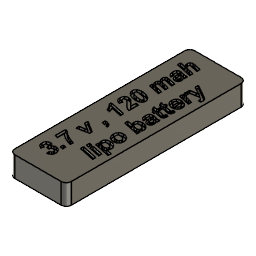
Battery (Autodesk Fusion 360 design; units mm, degrees)
part number: 2026-07-18-00-20-30-894
Autodesk Fusion 360 part; units mm, degrees
sketch "Sketch1" plane through (0, 0, 0) normal (0, 0, 1) x (1, 0, 0)
  line L0 (-49, 45) -> (-40, 45)
  line L1 (-39, 44) -> (-39, 11)
  line L2 (-40, 10) -> (-49, 10)
  line L3 (-50, 11) -> (-50, 44)
  arc A0 (-49, 45) -> (-50, 44) centre (-49, 44) ccw
  arc A1 (-39, 44) -> (-40, 45) centre (-40, 44) ccw
  arc A2 (-40, 10) -> (-39, 11) centre (-40, 11) ccw
  arc A3 (-50, 11) -> (-49, 10) centre (-49, 11) ccw
  point P0 (-50, 45)
  point P1 (-39, 45)
  point P2 (-50, 10)
  dimension "d3" = 11
  dimension "d4" = 35
  dimension "d5" = 1
  constraint perpendicular L0 L1
  constraint parallel L0 L2
  constraint parallel L1 L3
  constraint horizontal L0
  constraint coincident P0 L0
  constraint coincident P0 L3
  constraint tangent L0 A0
  constraint tangent L3 A0
  constraint coincident P1 L0
  constraint coincident P1 L1
  constraint tangent L0 A1
  constraint tangent L1 A1
  constraint equal A0 A1
  constraint tangent L1 A2
  constraint tangent L2 A2
  constraint equal A0 A2
  constraint coincident P2 L2
  constraint coincident P2 L3
  constraint tangent L2 A3
  constraint tangent L3 A3
  constraint equal A0 A3
  measures "d3" distance of P0 P1
  measures "d4" distance of P0 P2
  measures "d5" radius of A0
extrude "Extrude1" add sketch "Sketch1" along normal blind 4
sketch "Sketch2" plane through (0, 0, 4) normal (0, 0, 1) x (-1, 0, 0)
  arc A0 (49, -45) -> (50, -44) centre (49, -44) ccw
  line L0 (50, -44) -> (50, -11)
  arc A1 (50, -11) -> (49, -10) centre (49, -11) ccw
  line L1 (49, -10) -> (40, -10)
  arc A2 (40, -10) -> (39, -11) centre (40, -11) ccw
  line L2 (39, -11) -> (39, -44)
  arc A3 (39, -44) -> (40, -45) centre (40, -44) ccw
  line L3 (40, -45) -> (49, -45)
  line L4 (46.1248, -13.354) -> (46.1924, -13.9168)
  spline S0 degree 2 poles (46.1924, -13.9168) (45.9529, -13.9516) (45.8608, -14.0426) knots 0 0 0 1 1 1
  spline S1 degree 2 poles (45.8608, -14.0426) (45.7688, -14.1337) (45.7688, -14.2851) knots 0 0 0 1 1 1
  spline S2 degree 2 poles (45.7688, -14.2851) (45.7688, -14.4857) (45.9038, -14.6177) knots 0 0 0 1 1 1
  spline S3 degree 2 poles (45.9038, -14.6177) (46.0389, -14.7497) (46.2497, -14.7497) knots 0 0 0 1 1 1
  spline S4 degree 2 poles (46.2497, -14.7497) (46.4338, -14.7497) (46.5413, -14.6432) knots 0 0 0 1 1 1
  spline S5 degree 2 poles (46.5413, -14.6432) (46.6487, -14.5368) (46.6487, -14.3568) knots 0 0 0 1 1 1
  spline S6 degree 2 poles (46.6487, -14.3568) (46.6487, -14.3117) (46.6405, -14.2626) knots 0 0 0 1 1 1
  line L5 (46.6405, -14.2626) -> (47.1296, -14.3649)
  spline S7 degree 2 poles (47.1296, -14.3649) (47.1255, -14.3956) (47.1255, -14.4243) knots 0 0 0 1 1 1
  spline S8 degree 2 poles (47.1255, -14.4243) (47.1255, -14.6596) (47.2452, -14.7824) knots 0 0 0 1 1 1
  spline S9 degree 2 poles (47.2452, -14.7824) (47.3649, -14.9052) (47.5696, -14.9052) knots 0 0 0 1 1 1
  spline S10 degree 2 poles (47.5696, -14.9052) (47.7149, -14.9052) (47.7988, -14.8223) knots 0 0 0 1 1 1
  spline S11 degree 2 poles (47.7988, -14.8223) (47.8827, -14.7394) (47.8827, -14.6044) knots 0 0 0 1 1 1
  spline S12 degree 2 poles (47.8827, -14.6044) (47.8827, -14.4775) (47.7896, -14.3772) knots 0 0 0 1 1 1
  spline S13 degree 2 poles (47.7896, -14.3772) (47.6965, -14.2769) (47.4714, -14.2176) knots 0 0 0 1 1 1
  line L6 (47.4714, -14.2176) -> (47.5778, -13.6814)
  spline S14 degree 2 poles (47.5778, -13.6814) (47.9093, -13.7838) (48.0873, -13.9659) knots 0 0 0 1 1 1
  spline S15 degree 2 poles (48.0873, -13.9659) (48.3533, -14.2422) (48.3533, -14.6453) knots 0 0 0 1 1 1
  spline S16 degree 2 poles (48.3533, -14.6453) (48.3533, -15.0587) (48.1231, -15.2735) knots 0 0 0 1 1 1
  spline S17 degree 2 poles (48.1231, -15.2735) (47.8929, -15.4884) (47.5716, -15.4884) knots 0 0 0 1 1 1
  spline S18 degree 2 poles (47.5716, -15.4884) (47.3383, -15.4884) (47.1501, -15.3513) knots 0 0 0 1 1 1
  spline S19 degree 2 poles (47.1501, -15.3513) (46.9618, -15.2142) (46.8738, -14.9748) knots 0 0 0 1 1 1
  spline S20 degree 2 poles (46.8738, -14.9748) (46.7735, -15.1651) (46.6139, -15.2551) knots 0 0 0 1 1 1
  spline S21 degree 2 poles (46.6139, -15.2551) (46.4543, -15.3452) (46.2804, -15.3452) knots 0 0 0 1 1 1
  spline S22 degree 2 poles (46.2804, -15.3452) (45.9488, -15.3452) (45.6705, -15.1098) knots 0 0 0 1 1 1
  spline S23 degree 2 poles (45.6705, -15.1098) (45.2899, -14.7885) (45.2899, -14.281) knots 0 0 0 1 1 1
  spline S24 degree 2 poles (45.2899, -14.281) (45.2899, -13.9004) (45.5078, -13.6538) knots 0 0 0 1 1 1
  spline S25 degree 2 poles (45.5078, -13.6538) (45.7258, -13.4072) (46.1248, -13.354) knots 0 0 0 1 1 1
  line L7 (45.9079, -15.7749) -> (45.9079, -16.3561)
  line L8 (45.9079, -16.3561) -> (45.3411, -16.2374)
  line L9 (45.3411, -16.2374) -> (45.3411, -15.6562)
  line L10 (45.3411, -15.6562) -> (45.9079, -15.7749)
  line L11 (47.7578, -17.0703) -> (48.3001, -17.1828)
  line L12 (48.3001, -17.1828) -> (48.3001, -19.1617)
  line L13 (48.3001, -19.1617) -> (47.8827, -19.0737)
  spline S26 degree 2 poles (47.8827, -19.0737) (47.7312, -18.8854) (47.4274, -18.6583) knots 0 0 0 1 1 1
  spline S27 degree 2 poles (47.4274, -18.6583) (47.1235, -18.4311) (46.748, -18.2377) knots 0 0 0 1 1 1
  spline S28 degree 2 poles (46.748, -18.2377) (46.3724, -18.0443) (46.0348, -17.9216) knots 0 0 0 1 1 1
  spline S29 degree 2 poles (46.0348, -17.9216) (45.5682, -17.7517) (45.3411, -17.7108) knots 0 0 0 1 1 1
  line L14 (45.3411, -17.7108) -> (45.3411, -17.1521)
  spline S30 degree 2 poles (45.3411, -17.1521) (45.5662, -17.189) (45.9591, -17.3261) knots 0 0 0 1 1 1
  spline S31 degree 2 poles (45.9591, -17.3261) (46.442, -17.4939) (46.8922, -17.7456) knots 0 0 0 1 1 1
  spline S32 degree 2 poles (46.8922, -17.7456) (47.3424, -17.9973) (47.7578, -18.3533) knots 0 0 0 1 1 1
  line L15 (47.7578, -18.3533) -> (47.7578, -17.0703)
  line L16 (45.3411, -21.3861) -> (45.3411, -20.8806)
  line L17 (45.3411, -20.8806) -> (47.5143, -20.4447)
  line L18 (47.5143, -20.4447) -> (47.5143, -21.0218)
  line L19 (47.5143, -21.0218) -> (46.5668, -21.1753)
  spline S33 degree 2 poles (46.5668, -21.1753) (46.1821, -21.2387) (46.0553, -21.251) knots 0 0 0 1 1 1
  spline S34 degree 2 poles (46.0553, -21.251) (46.09, -21.2674) (46.3203, -21.3932) knots 0 0 0 1 1 1
  spline S35 degree 2 poles (46.3203, -21.3932) (46.5505, -21.5191) (46.5975, -21.5478) knots 0 0 0 1 1 1
  line L20 (46.5975, -21.5478) -> (47.5143, -22.088)
  line L21 (47.5143, -22.088) -> (47.5143, -22.7224)
  line L22 (47.5143, -22.7224) -> (45.3411, -21.3861)
  line L23 (45.9079, -23.9256) -> (45.9079, -24.5171)
  line L24 (45.9079, -24.5171) -> (45.4393, -24.4188)
  spline S36 degree 2 poles (45.4393, -24.4188) (45.0341, -24.3349) (44.8653, -24.1497) knots 0 0 0 1 1 1
  spline S37 degree 2 poles (44.8653, -24.1497) (44.6965, -23.9645) (44.6903, -23.6699) knots 0 0 0 1 1 1
  line L25 (44.6903, -23.6699) -> (44.9625, -23.7271)
  spline S38 degree 2 poles (44.9625, -23.7271) (44.9952, -23.8745) (45.0802, -23.9553) knots 0 0 0 1 1 1
  spline S39 degree 2 poles (45.0802, -23.9553) (45.1651, -24.0362) (45.3411, -24.075) knots 0 0 0 1 1 1
  line L26 (45.3411, -24.075) -> (45.3411, -23.8049)
  line L27 (45.3411, -23.8049) -> (45.9079, -23.9256)
  line L28 (47.0641, -26.4529) -> (47.588, -26.5634)
  spline S40 degree 2 poles (47.588, -26.5634) (47.9195, -27.3226) (48.3595, -27.7381) knots 0 0 0 1 1 1
  line L29 (48.3595, -27.7381) -> (48.3595, -28.0962)
  line L30 (48.3595, -28.0962) -> (45.3411, -27.4638)
  line L31 (45.3411, -27.4638) -> (45.3411, -26.8724)
  line L32 (45.3411, -26.8724) -> (47.4202, -27.3083)
  spline S41 degree 2 poles (47.4202, -27.3083) (47.3015, -27.1241) (47.2033, -26.8837) knots 0 0 0 1 1 1
  spline S42 degree 2 poles (47.2033, -26.8837) (47.105, -26.6432) (47.0641, -26.4529) knots 0 0 0 1 1 1
  line L33 (47.4059, -29.3936) -> (47.4918, -28.8186)
  spline S43 degree 2 poles (47.4918, -28.8186) (47.9093, -28.8881) (48.1313, -29.1429) knots 0 0 0 1 1 1
  spline S44 degree 2 poles (48.1313, -29.1429) (48.3533, -29.3977) (48.3533, -29.7804) knots 0 0 0 1 1 1
  spline S45 degree 2 poles (48.3533, -29.7804) (48.3533, -30.1999) (48.1262, -30.4393) knots 0 0 0 1 1 1
  spline S46 degree 2 poles (48.1262, -30.4393) (47.899, -30.6787) (47.5491, -30.6787) knots 0 0 0 1 1 1
  spline S47 degree 2 poles (47.5491, -30.6787) (47.3711, -30.6787) (47.192, -30.605) knots 0 0 0 1 1 1
  spline S48 degree 2 poles (47.192, -30.605) (47.013, -30.5314) (46.8165, -30.3636) knots 0 0 0 1 1 1
  spline S49 degree 2 poles (46.8165, -30.3636) (46.6774, -30.2428) (46.4226, -29.9686) knots 0 0 0 1 1 1
  spline S50 degree 2 poles (46.4226, -29.9686) (46.1678, -29.6944) (46.0747, -29.6054) knots 0 0 0 1 1 1
  spline S51 degree 2 poles (46.0747, -29.6054) (45.9816, -29.5164) (45.8772, -29.4345) knots 0 0 0 1 1 1
  line L34 (45.8772, -29.4345) -> (45.8772, -30.4741)
  line L35 (45.8772, -30.4741) -> (45.3411, -30.3636)
  line L36 (45.3411, -30.3636) -> (45.3411, -28.5402)
  spline S52 degree 2 poles (45.3411, -28.5402) (45.5621, -28.5689) (45.7616, -28.6702) knots 0 0 0 1 1 1
  spline S53 degree 2 poles (45.7616, -28.6702) (45.9611, -28.7715) (46.133, -28.9229) knots 0 0 0 1 1 1
  spline S54 degree 2 poles (46.133, -28.9229) (46.3049, -29.0744) (46.6876, -29.4775) knots 0 0 0 1 1 1
  spline S55 degree 2 poles (46.6876, -29.4775) (46.9782, -29.7804) (47.0662, -29.8602) knots 0 0 0 1 1 1
  spline S56 degree 2 poles (47.0662, -29.8602) (47.2258, -30.0034) (47.3424, -30.0566) knots 0 0 0 1 1 1
  spline S57 degree 2 poles (47.3424, -30.0566) (47.4591, -30.1098) (47.5532, -30.1098) knots 0 0 0 1 1 1
  spline S58 degree 2 poles (47.5532, -30.1098) (47.7046, -30.1098) (47.7988, -30.0208) knots 0 0 0 1 1 1
  spline S59 degree 2 poles (47.7988, -30.0208) (47.8929, -29.9318) (47.8929, -29.7947) knots 0 0 0 1 1 1
  spline S60 degree 2 poles (47.8929, -29.7947) (47.8929, -29.6555) (47.7875, -29.5512) knots 0 0 0 1 1 1
  spline S61 degree 2 poles (47.7875, -29.5512) (47.6821, -29.4468) (47.4059, -29.3936) knots 0 0 0 1 1 1
  spline S62 degree 2 poles (46.3172, -30.8874) (46.7694, -30.8874) (47.234, -31.0409) knots 0 0 0 1 1 1
  spline S63 degree 2 poles (47.234, -31.0409) (47.8008, -31.2292) (48.0771, -31.5239) knots 0 0 0 1 1 1
  spline S64 degree 2 poles (48.0771, -31.5239) (48.3533, -31.8186) (48.3533, -32.1787) knots 0 0 0 1 1 1
  spline S65 degree 2 poles (48.3533, -32.1787) (48.3533, -32.543) (48.0894, -32.7773) knots 0 0 0 1 1 1
  spline S66 degree 2 poles (48.0894, -32.7773) (47.8254, -33.0116) (47.322, -33.0116) knots 0 0 0 1 1 1
  spline S67 degree 2 poles (47.322, -33.0116) (46.8615, -33.0116) (46.3489, -32.8407) knots 0 0 0 1 1 1
  spline S68 degree 2 poles (46.3489, -32.8407) (45.8363, -32.6699) (45.5631, -32.3793) knots 0 0 0 1 1 1
  spline S69 degree 2 poles (45.5631, -32.3793) (45.2899, -32.0887) (45.2899, -31.7244) knots 0 0 0 1 1 1
  spline S70 degree 2 poles (45.2899, -31.7244) (45.2899, -31.3602) (45.5539, -31.1238) knots 0 0 0 1 1 1
  spline S71 degree 2 poles (45.5539, -31.1238) (45.8179, -30.8874) (46.3172, -30.8874) knots 0 0 0 1 1 1
  spline S72 degree 2 poles (46.1985, -31.4645) (45.957, -31.4645) (45.8588, -31.5423) knots 0 0 0 1 1 1
  spline S73 degree 2 poles (45.8588, -31.5423) (45.7606, -31.6201) (45.7606, -31.7428) knots 0 0 0 1 1 1
  spline S74 degree 2 poles (45.7606, -31.7428) (45.7606, -31.9065) (45.912, -32.0334) knots 0 0 0 1 1 1
  spline S75 degree 2 poles (45.912, -32.0334) (46.1146, -32.2033) (46.7101, -32.3342) knots 0 0 0 1 1 1
  spline S76 degree 2 poles (46.7101, -32.3342) (47.1828, -32.4386) (47.4591, -32.4386) knots 0 0 0 1 1 1
  spline S77 degree 2 poles (47.4591, -32.4386) (47.6842, -32.4386) (47.7834, -32.3598) knots 0 0 0 1 1 1
  spline S78 degree 2 poles (47.7834, -32.3598) (47.8827, -32.281) (47.8827, -32.1583) knots 0 0 0 1 1 1
  spline S79 degree 2 poles (47.8827, -32.1583) (47.8827, -32.0027) (47.7333, -31.882) knots 0 0 0 1 1 1
  spline S80 degree 2 poles (47.7333, -31.882) (47.5164, -31.704) (46.97, -31.575) knots 0 0 0 1 1 1
  spline S81 degree 2 poles (46.97, -31.575) (46.4973, -31.4645) (46.1985, -31.4645) knots 0 0 0 1 1 1
  line L37 (47.5143, -34.7162) -> (47.5143, -35.2688)
  line L38 (47.5143, -35.2688) -> (47.2503, -35.2135)
  spline S82 degree 2 poles (47.2503, -35.2135) (47.5655, -35.5368) (47.5655, -35.8929) knots 0 0 0 1 1 1
  spline S83 degree 2 poles (47.5655, -35.8929) (47.5655, -36.1385) (47.4632, -36.2715) knots 0 0 0 1 1 1
  spline S84 degree 2 poles (47.4632, -36.2715) (47.3608, -36.4045) (47.1808, -36.4413) knots 0 0 0 1 1 1
  spline S85 degree 2 poles (47.1808, -36.4413) (47.3445, -36.5539) (47.455, -36.7647) knots 0 0 0 1 1 1
  spline S86 degree 2 poles (47.455, -36.7647) (47.5655, -36.9754) (47.5655, -37.2026) knots 0 0 0 1 1 1
  spline S87 degree 2 poles (47.5655, -37.2026) (47.5655, -37.4625) (47.4263, -37.6078) knots 0 0 0 1 1 1
  spline S88 degree 2 poles (47.4263, -37.6078) (47.2872, -37.7531) (47.058, -37.7531) knots 0 0 0 1 1 1
  spline S89 degree 2 poles (47.058, -37.7531) (46.9454, -37.7531) (46.6692, -37.6958) knots 0 0 0 1 1 1
  line L39 (46.6692, -37.6958) -> (45.3411, -37.4175)
  line L40 (45.3411, -37.4175) -> (45.3411, -36.8302)
  line L41 (45.3411, -36.8302) -> (46.6692, -37.1085)
  spline S90 degree 2 poles (46.6692, -37.1085) (46.9188, -37.1596) (46.9516, -37.1596) knots 0 0 0 1 1 1
  spline S91 degree 2 poles (46.9516, -37.1596) (47.0416, -37.1596) (47.0938, -37.1054) knots 0 0 0 1 1 1
  spline S92 degree 2 poles (47.0938, -37.1054) (47.146, -37.0512) (47.146, -36.9427) knots 0 0 0 1 1 1
  spline S93 degree 2 poles (47.146, -36.9427) (47.146, -36.7237) (46.9147, -36.5518) knots 0 0 0 1 1 1
  spline S94 degree 2 poles (46.9147, -36.5518) (46.749, -36.427) (46.3274, -36.339) knots 0 0 0 1 1 1
  line L42 (46.3274, -36.339) -> (45.3411, -36.1323)
  line L43 (45.3411, -36.1323) -> (45.3411, -35.545)
  line L44 (45.3411, -35.545) -> (46.6548, -35.8192)
  spline S95 degree 2 poles (46.6548, -35.8192) (46.882, -35.8663) (46.9495, -35.8663) knots 0 0 0 1 1 1
  spline S96 degree 2 poles (46.9495, -35.8663) (47.0355, -35.8663) (47.0907, -35.808) knots 0 0 0 1 1 1
  spline S97 degree 2 poles (47.0907, -35.808) (47.146, -35.7497) (47.146, -35.6473) knots 0 0 0 1 1 1
  spline S98 degree 2 poles (47.146, -35.6473) (47.146, -35.5512) (47.0887, -35.4488) knots 0 0 0 1 1 1
  spline S99 degree 2 poles (47.0887, -35.4488) (47.0314, -35.3465) (46.9311, -35.2698) knots 0 0 0 1 1 1
  spline S100 degree 2 poles (46.9311, -35.2698) (46.8308, -35.193) (46.6733, -35.1378) knots 0 0 0 1 1 1
  spline S101 degree 2 poles (46.6733, -35.1378) (46.5996, -35.1132) (46.3397, -35.058) knots 0 0 0 1 1 1
  line L45 (46.3397, -35.058) -> (45.3411, -34.8493)
  line L46 (45.3411, -34.8493) -> (45.3411, -34.2619)
  line L47 (45.3411, -34.2619) -> (47.5143, -34.7162)
  line L48 (46.8984, -38.8356) -> (46.9475, -38.2626)
  spline S102 degree 2 poles (46.9475, -38.2626) (47.2381, -38.3608) (47.4018, -38.6054) knots 0 0 0 1 1 1
  spline S103 degree 2 poles (47.4018, -38.6054) (47.5655, -38.8499) (47.5655, -39.2531) knots 0 0 0 1 1 1
  spline S104 degree 2 poles (47.5655, -39.2531) (47.5655, -39.6726) (47.3967, -39.8731) knots 0 0 0 1 1 1
  spline S105 degree 2 poles (47.3967, -39.8731) (47.2278, -40.0737) (46.9843, -40.0737) knots 0 0 0 1 1 1
  spline S106 degree 2 poles (46.9843, -40.0737) (46.8861, -40.0737) (46.7756, -40.0563) knots 0 0 0 1 1 1
  spline S107 degree 2 poles (46.7756, -40.0563) (46.6651, -40.0389) (46.1944, -39.9345) knots 0 0 0 1 1 1
  spline S108 degree 2 poles (46.1944, -39.9345) (45.8056, -39.8486) (45.6501, -39.8486) knots 0 0 0 1 1 1
  spline S109 degree 2 poles (45.6501, -39.8486) (45.5109, -39.8486) (45.3411, -39.8977) knots 0 0 0 1 1 1
  line L49 (45.3411, -39.8977) -> (45.3411, -39.3267)
  spline S110 degree 2 poles (45.3411, -39.3267) (45.4598, -39.292) (45.5866, -39.2838) knots 0 0 0 1 1 1
  spline S111 degree 2 poles (45.5866, -39.2838) (45.4434, -39.1548) (45.3666, -38.987) knots 0 0 0 1 1 1
  spline S112 degree 2 poles (45.3666, -38.987) (45.2899, -38.8192) (45.2899, -38.6494) knots 0 0 0 1 1 1
  spline S113 degree 2 poles (45.2899, -38.6494) (45.2899, -38.3793) (45.4669, -38.2033) knots 0 0 0 1 1 1
  spline S114 degree 2 poles (45.4669, -38.2033) (45.6439, -38.0273) (45.9222, -38.0273) knots 0 0 0 1 1 1
  spline S115 degree 2 poles (45.9222, -38.0273) (46.2333, -38.0273) (46.4195, -38.2207) knots 0 0 0 1 1 1
  spline S116 degree 2 poles (46.4195, -38.2207) (46.6057, -38.4141) (46.6446, -38.9113) knots 0 0 0 1 1 1
  spline S117 degree 2 poles (46.6446, -38.9113) (46.6794, -39.3308) (46.7285, -39.472) knots 0 0 0 1 1 1
  spline S118 degree 2 poles (46.7285, -39.472) (46.8513, -39.5089) (46.925, -39.5089) knots 0 0 0 1 1 1
  spline S119 degree 2 poles (46.925, -39.5089) (47.0191, -39.5089) (47.0825, -39.4332) knots 0 0 0 1 1 1
  spline S120 degree 2 poles (47.0825, -39.4332) (47.146, -39.3574) (47.146, -39.2081) knots 0 0 0 1 1 1
  spline S121 degree 2 poles (47.146, -39.2081) (47.146, -39.0505) (47.0815, -38.9594) knots 0 0 0 1 1 1
  spline S122 degree 2 poles (47.0815, -38.9594) (47.0171, -38.8684) (46.8984, -38.8356) knots 0 0 0 1 1 1
  spline S123 degree 2 poles (46.354, -39.3943) (46.3397, -39.3411) (46.3274, -39.2531) knots 0 0 0 1 1 1
  spline S124 degree 2 poles (46.3274, -39.2531) (46.2742, -38.8111) (46.1719, -38.676) knots 0 0 0 1 1 1
  spline S125 degree 2 poles (46.1719, -38.676) (46.0982, -38.5798) (45.9734, -38.5798) knots 0 0 0 1 1 1
  spline S126 degree 2 poles (45.9734, -38.5798) (45.8711, -38.5798) (45.8005, -38.6535) knots 0 0 0 1 1 1
  spline S127 degree 2 poles (45.8005, -38.6535) (45.7299, -38.7272) (45.7299, -38.8479) knots 0 0 0 1 1 1
  spline S128 degree 2 poles (45.7299, -38.8479) (45.7299, -38.9809) (45.7943, -39.0986) knots 0 0 0 1 1 1
  spline S129 degree 2 poles (45.7943, -39.0986) (45.8588, -39.2162) (45.9601, -39.2746) knots 0 0 0 1 1 1
  spline S130 degree 2 poles (45.9601, -39.2746) (46.0614, -39.3329) (46.2763, -39.3779) knots 0 0 0 1 1 1
  line L50 (46.2763, -39.3779) -> (46.354, -39.3943)
  line L51 (45.3411, -40.9332) -> (45.3411, -40.3458)
  line L52 (45.3411, -40.3458) -> (48.3411, -40.9741)
  line L53 (48.3411, -40.9741) -> (48.3411, -41.5614)
  line L54 (48.3411, -41.5614) -> (47.2729, -41.3363)
  spline S131 degree 2 poles (47.2729, -41.3363) (47.4284, -41.5348) (47.4969, -41.7067) knots 0 0 0 1 1 1
  spline S132 degree 2 poles (47.4969, -41.7067) (47.5655, -41.8786) (47.5655, -42.075) knots 0 0 0 1 1 1
  spline S133 degree 2 poles (47.5655, -42.075) (47.5655, -42.339) (47.4141, -42.4925) knots 0 0 0 1 1 1
  spline S134 degree 2 poles (47.4141, -42.4925) (47.2626, -42.646) (47.0171, -42.646) knots 0 0 0 1 1 1
  spline S135 degree 2 poles (47.0171, -42.646) (46.8861, -42.646) (46.6119, -42.5887) knots 0 0 0 1 1 1
  line L55 (46.6119, -42.5887) -> (45.3411, -42.3226)
  line L56 (45.3411, -42.3226) -> (45.3411, -41.7353)
  line L57 (45.3411, -41.7353) -> (46.6364, -42.0075)
  spline S136 degree 2 poles (46.6364, -42.0075) (46.8472, -42.0505) (46.9065, -42.0505) knots 0 0 0 1 1 1
  spline S137 degree 2 poles (46.9065, -42.0505) (47.015, -42.0505) (47.0805, -41.9829) knots 0 0 0 1 1 1
  spline S138 degree 2 poles (47.0805, -41.9829) (47.146, -41.9154) (47.146, -41.7988) knots 0 0 0 1 1 1
  spline S139 degree 2 poles (47.146, -41.7988) (47.146, -41.6514) (47.0437, -41.5164) knots 0 0 0 1 1 1
  spline S140 degree 2 poles (47.0437, -41.5164) (46.9086, -41.3404) (46.7121, -41.2483) knots 0 0 0 1 1 1
  spline S141 degree 2 poles (46.7121, -41.2483) (46.6037, -41.1971) (46.2026, -41.1132) knots 0 0 0 1 1 1
  line L58 (46.2026, -41.1132) -> (45.3411, -40.9332)
  line L59 (40.6589, -16.8053) -> (43.6589, -17.4335)
  line L60 (43.6589, -17.4335) -> (43.6589, -18.0188)
  line L61 (43.6589, -18.0188) -> (40.6589, -17.3926)
  line L62 (40.6589, -17.3926) -> (40.6589, -16.8053)
  line L63 (43.6589, -18.5999) -> (43.6589, -19.1872)
  line L64 (43.6589, -19.1872) -> (43.1269, -19.0767)
  line L65 (43.1269, -19.0767) -> (43.1269, -18.4894)
  line L66 (43.1269, -18.4894) -> (43.6589, -18.5999)
  line L67 (42.8322, -18.428) -> (42.8322, -19.0153)
  line L68 (42.8322, -19.0153) -> (40.6589, -18.5611)
  line L69 (40.6589, -18.5611) -> (40.6589, -17.9737)
  line L70 (40.6589, -17.9737) -> (42.8322, -18.428)
  line L71 (42.8322, -19.574) -> (42.8322, -20.1306)
  line L72 (42.8322, -20.1306) -> (42.6091, -20.0836)
  spline S142 degree 2 poles (42.6091, -20.0836) (42.7565, -20.2616) (42.8199, -20.4171) knots 0 0 0 1 1 1
  spline S143 degree 2 poles (42.8199, -20.4171) (42.8834, -20.5726) (42.8834, -20.7507) knots 0 0 0 1 1 1
  spline S144 degree 2 poles (42.8834, -20.7507) (42.8834, -21.0924) (42.648, -21.3001) knots 0 0 0 1 1 1
  spline S145 degree 2 poles (42.648, -21.3001) (42.4127, -21.5078) (41.9461, -21.5078) knots 0 0 0 1 1 1
  spline S146 degree 2 poles (41.9461, -21.5078) (41.3588, -21.5078) (40.9536, -21.1497) knots 0 0 0 1 1 1
  spline S147 degree 2 poles (40.9536, -21.1497) (40.6078, -20.8428) (40.6078, -20.4233) knots 0 0 0 1 1 1
  spline S148 degree 2 poles (40.6078, -20.4233) (40.6078, -19.9915) (40.9577, -19.7705) knots 0 0 0 1 1 1
  line L73 (40.9577, -19.7705) -> (39.8302, -19.5351)
  line L74 (39.8302, -19.5351) -> (39.8302, -18.9478)
  line L75 (39.8302, -18.9478) -> (42.8322, -19.574)
  spline S149 degree 2 poles (41.5859, -19.928) (41.3322, -19.928) (41.192, -20.0518) knots 0 0 0 1 1 1
  spline S150 degree 2 poles (41.192, -20.0518) (41.0518, -20.1756) (41.0518, -20.3435) knots 0 0 0 1 1 1
  spline S151 degree 2 poles (41.0518, -20.3435) (41.0518, -20.4887) (41.1572, -20.6238) knots 0 0 0 1 1 1
  spline S152 degree 2 poles (41.1572, -20.6238) (41.2626, -20.7589) (41.5072, -20.8479) knots 0 0 0 1 1 1
  spline S153 degree 2 poles (41.5072, -20.8479) (41.7517, -20.9369) (41.9604, -20.9369) knots 0 0 0 1 1 1
  spline S154 degree 2 poles (41.9604, -20.9369) (42.204, -20.9369) (42.3339, -20.8203) knots 0 0 0 1 1 1
  spline S155 degree 2 poles (42.3339, -20.8203) (42.4638, -20.7036) (42.4638, -20.5235) knots 0 0 0 1 1 1
  spline S156 degree 2 poles (42.4638, -20.5235) (42.4638, -20.3557) (42.3441, -20.2176) knots 0 0 0 1 1 1
  spline S157 degree 2 poles (42.3441, -20.2176) (42.2244, -20.0795) (41.9922, -20.0038) knots 0 0 0 1 1 1
  spline S158 degree 2 poles (41.9922, -20.0038) (41.7599, -19.928) (41.5859, -19.928) knots 0 0 0 1 1 1
  spline S159 degree 2 poles (41.5614, -21.7841) (42.1651, -21.7841) (42.5242, -22.1248) knots 0 0 0 1 1 1
  spline S160 degree 2 poles (42.5242, -22.1248) (42.8834, -22.4656) (42.8834, -23.0201) knots 0 0 0 1 1 1
  spline S161 degree 2 poles (42.8834, -23.0201) (42.8834, -23.501) (42.6183, -23.7711) knots 0 0 0 1 1 1
  spline S162 degree 2 poles (42.6183, -23.7711) (42.3533, -24.0413) (41.9052, -24.0413) knots 0 0 0 1 1 1
  spline S163 degree 2 poles (41.9052, -24.0413) (41.3772, -24.0413) (40.9925, -23.7036) knots 0 0 0 1 1 1
  spline S164 degree 2 poles (40.9925, -23.7036) (40.6078, -23.366) (40.6078, -22.7991) knots 0 0 0 1 1 1
  spline S165 degree 2 poles (40.6078, -22.7991) (40.6078, -22.4922) (40.7306, -22.2548) knots 0 0 0 1 1 1
  spline S166 degree 2 poles (40.7306, -22.2548) (40.8533, -22.0174) (41.0784, -21.9008) knots 0 0 0 1 1 1
  spline S167 degree 2 poles (41.0784, -21.9008) (41.3035, -21.7841) (41.5614, -21.7841) knots 0 0 0 1 1 1
  spline S168 degree 2 poles (41.9809, -23.458) (42.1896, -23.458) (42.3155, -23.3363) knots 0 0 0 1 1 1
  spline S169 degree 2 poles (42.3155, -23.3363) (42.4413, -23.2145) (42.4413, -23.0222) knots 0 0 0 1 1 1
  spline S170 degree 2 poles (42.4413, -23.0222) (42.4413, -22.8319) (42.3237, -22.6845) knots 0 0 0 1 1 1
  spline S171 degree 2 poles (42.3237, -22.6845) (42.206, -22.5372) (41.9819, -22.4553) knots 0 0 0 1 1 1
  spline S172 degree 2 poles (41.9819, -22.4553) (41.7578, -22.3735) (41.5696, -22.3735) knots 0 0 0 1 1 1
  spline S173 degree 2 poles (41.5696, -22.3735) (41.3363, -22.3735) (41.1992, -22.5003) knots 0 0 0 1 1 1
  spline S174 degree 2 poles (41.1992, -22.5003) (41.0621, -22.6272) (41.0621, -22.8196) knots 0 0 0 1 1 1
  spline S175 degree 2 poles (41.0621, -22.8196) (41.0621, -23.061) (41.2688, -23.2248) knots 0 0 0 1 1 1
  spline S176 degree 2 poles (41.2688, -23.2248) (41.5614, -23.458) (41.9809, -23.458) knots 0 0 0 1 1 1
  line L76 (40.6589, -25.4062) -> (43.6589, -26.0324)
  line L77 (43.6589, -26.0324) -> (43.6589, -26.6218)
  line L78 (43.6589, -26.6218) -> (42.6562, -26.411)
  spline S177 degree 2 poles (42.6562, -26.411) (42.779, -26.5726) (42.8312, -26.7128) knots 0 0 0 1 1 1
  spline S178 degree 2 poles (42.8312, -26.7128) (42.8834, -26.853) (42.8834, -27.0188) knots 0 0 0 1 1 1
  spline S179 degree 2 poles (42.8834, -27.0188) (42.8834, -27.3626) (42.6531, -27.5692) knots 0 0 0 1 1 1
  spline S180 degree 2 poles (42.6531, -27.5692) (42.4229, -27.7759) (41.9829, -27.7759) knots 0 0 0 1 1 1
  spline S181 degree 2 poles (41.9829, -27.7759) (41.6862, -27.7759) (41.4069, -27.6787) knots 0 0 0 1 1 1
  spline S182 degree 2 poles (41.4069, -27.6787) (41.1276, -27.5815) (40.9526, -27.4188) knots 0 0 0 1 1 1
  spline S183 degree 2 poles (40.9526, -27.4188) (40.7776, -27.2561) (40.6927, -27.0771) knots 0 0 0 1 1 1
  spline S184 degree 2 poles (40.6927, -27.0771) (40.6078, -26.898) (40.6078, -26.7016) knots 0 0 0 1 1 1
  spline S185 degree 2 poles (40.6078, -26.7016) (40.6078, -26.235) (41.0171, -26.016) knots 0 0 0 1 1 1
  line L79 (41.0171, -26.016) -> (40.6589, -25.9403)
  line L80 (40.6589, -25.9403) -> (40.6589, -25.4062)
  spline S186 degree 2 poles (41.545, -26.1982) (41.3261, -26.1982) (41.189, -26.322) knots 0 0 0 1 1 1
  spline S187 degree 2 poles (41.189, -26.322) (41.0518, -26.4458) (41.0518, -26.6136) knots 0 0 0 1 1 1
  spline S188 degree 2 poles (41.0518, -26.6136) (41.0518, -26.7609) (41.1583, -26.895) knots 0 0 0 1 1 1
  spline S189 degree 2 poles (41.1583, -26.895) (41.2647, -27.029) (41.498, -27.118) knots 0 0 0 1 1 1
  spline S190 degree 2 poles (41.498, -27.118) (41.7312, -27.207) (41.9686, -27.207) knots 0 0 0 1 1 1
  spline S191 degree 2 poles (41.9686, -27.207) (42.1999, -27.207) (42.3319, -27.0873) knots 0 0 0 1 1 1
  spline S192 degree 2 poles (42.3319, -27.0873) (42.4638, -26.9676) (42.4638, -26.7977) knots 0 0 0 1 1 1
  spline S193 degree 2 poles (42.4638, -26.7977) (42.4638, -26.5767) (42.2592, -26.4171) knots 0 0 0 1 1 1
  spline S194 degree 2 poles (42.2592, -26.4171) (41.9789, -26.1982) (41.545, -26.1982) knots 0 0 0 1 1 1
  line L81 (42.2162, -28.8114) -> (42.2653, -28.2384)
  spline S195 degree 2 poles (42.2653, -28.2384) (42.5559, -28.3366) (42.7196, -28.5812) knots 0 0 0 1 1 1
  spline S196 degree 2 poles (42.7196, -28.5812) (42.8834, -28.8257) (42.8834, -29.2289) knots 0 0 0 1 1 1
  spline S197 degree 2 poles (42.8834, -29.2289) (42.8834, -29.6484) (42.7145, -29.8489) knots 0 0 0 1 1 1
  spline S198 degree 2 poles (42.7145, -29.8489) (42.5457, -30.0495) (42.3022, -30.0495) knots 0 0 0 1 1 1
  spline S199 degree 2 poles (42.3022, -30.0495) (42.204, -30.0495) (42.0935, -30.0321) knots 0 0 0 1 1 1
  spline S200 degree 2 poles (42.0935, -30.0321) (41.9829, -30.0147) (41.5123, -29.9103) knots 0 0 0 1 1 1
  spline S201 degree 2 poles (41.5123, -29.9103) (41.1235, -29.8244) (40.9679, -29.8244) knots 0 0 0 1 1 1
  spline S202 degree 2 poles (40.9679, -29.8244) (40.8288, -29.8244) (40.6589, -29.8735) knots 0 0 0 1 1 1
  line L82 (40.6589, -29.8735) -> (40.6589, -29.3025)
  spline S203 degree 2 poles (40.6589, -29.3025) (40.7776, -29.2677) (40.9045, -29.2595) knots 0 0 0 1 1 1
  spline S204 degree 2 poles (40.9045, -29.2595) (40.7613, -29.1306) (40.6845, -28.9628) knots 0 0 0 1 1 1
  spline S205 degree 2 poles (40.6845, -28.9628) (40.6078, -28.795) (40.6078, -28.6252) knots 0 0 0 1 1 1
  spline S206 degree 2 poles (40.6078, -28.6252) (40.6078, -28.355) (40.7848, -28.1791) knots 0 0 0 1 1 1
  spline S207 degree 2 poles (40.7848, -28.1791) (40.9618, -28.0031) (41.2401, -28.0031) knots 0 0 0 1 1 1
  spline S208 degree 2 poles (41.2401, -28.0031) (41.5512, -28.0031) (41.7374, -28.1965) knots 0 0 0 1 1 1
  spline S209 degree 2 poles (41.7374, -28.1965) (41.9236, -28.3898) (41.9625, -28.8871) knots 0 0 0 1 1 1
  spline S210 degree 2 poles (41.9625, -28.8871) (41.9973, -29.3066) (42.0464, -29.4478) knots 0 0 0 1 1 1
  spline S211 degree 2 poles (42.0464, -29.4478) (42.1692, -29.4847) (42.2428, -29.4847) knots 0 0 0 1 1 1
  spline S212 degree 2 poles (42.2428, -29.4847) (42.337, -29.4847) (42.4004, -29.4089) knots 0 0 0 1 1 1
  spline S213 degree 2 poles (42.4004, -29.4089) (42.4638, -29.3332) (42.4638, -29.1838) knots 0 0 0 1 1 1
  spline S214 degree 2 poles (42.4638, -29.1838) (42.4638, -29.0263) (42.3994, -28.9352) knots 0 0 0 1 1 1
  spline S215 degree 2 poles (42.3994, -28.9352) (42.3349, -28.8441) (42.2162, -28.8114) knots 0 0 0 1 1 1
  spline S216 degree 2 poles (41.6719, -29.3701) (41.6576, -29.3168) (41.6453, -29.2289) knots 0 0 0 1 1 1
  spline S217 degree 2 poles (41.6453, -29.2289) (41.5921, -28.7868) (41.4898, -28.6518) knots 0 0 0 1 1 1
  spline S218 degree 2 poles (41.4898, -28.6518) (41.4161, -28.5556) (41.2913, -28.5556) knots 0 0 0 1 1 1
  spline S219 degree 2 poles (41.2913, -28.5556) (41.189, -28.5556) (41.1184, -28.6293) knots 0 0 0 1 1 1
  spline S220 degree 2 poles (41.1184, -28.6293) (41.0477, -28.7029) (41.0477, -28.8237) knots 0 0 0 1 1 1
  spline S221 degree 2 poles (41.0477, -28.8237) (41.0477, -28.9567) (41.1122, -29.0744) knots 0 0 0 1 1 1
  spline S222 degree 2 poles (41.1122, -29.0744) (41.1767, -29.192) (41.278, -29.2503) knots 0 0 0 1 1 1
  spline S223 degree 2 poles (41.278, -29.2503) (41.3793, -29.3087) (41.5941, -29.3537) knots 0 0 0 1 1 1
  line L83 (41.5941, -29.3537) -> (41.6719, -29.3701)
  line L84 (42.3963, -30.4608) -> (42.8322, -30.5508)
  line L85 (42.8322, -30.5508) -> (42.8322, -30.8373)
  line L86 (42.8322, -30.8373) -> (43.1801, -30.9089)
  line L87 (43.1801, -30.9089) -> (43.5853, -31.5822)
  line L88 (43.5853, -31.5822) -> (42.8322, -31.4246)
  line L89 (42.8322, -31.4246) -> (42.8322, -31.7827)
  line L90 (42.8322, -31.7827) -> (42.3963, -31.6927)
  line L91 (42.3963, -31.6927) -> (42.3963, -31.3325)
  line L92 (42.3963, -31.3325) -> (41.4857, -31.1422)
  spline S224 degree 2 poles (41.4857, -31.1422) (41.2381, -31.0911) (41.2033, -31.0911) knots 0 0 0 1 1 1
  spline S225 degree 2 poles (41.2033, -31.0911) (41.1357, -31.0911) (41.0979, -31.134) knots 0 0 0 1 1 1
  spline S226 degree 2 poles (41.0979, -31.134) (41.06, -31.177) (41.06, -31.2896) knots 0 0 0 1 1 1
  spline S227 degree 2 poles (41.06, -31.2896) (41.06, -31.3284) (41.0744, -31.484) knots 0 0 0 1 1 1
  line L93 (41.0744, -31.484) -> (40.6385, -31.3919)
  spline S228 degree 2 poles (40.6385, -31.3919) (40.6078, -31.2404) (40.6078, -31.0808) knots 0 0 0 1 1 1
  spline S229 degree 2 poles (40.6078, -31.0808) (40.6078, -30.7698) (40.7275, -30.6286) knots 0 0 0 1 1 1
  spline S230 degree 2 poles (40.7275, -30.6286) (40.8472, -30.4874) (41.06, -30.4874) knots 0 0 0 1 1 1
  spline S231 degree 2 poles (41.06, -30.4874) (41.1603, -30.4874) (41.5225, -30.5631) knots 0 0 0 1 1 1
  line L94 (41.5225, -30.5631) -> (42.3963, -30.7452)
  line L95 (42.3963, -30.7452) -> (42.3963, -30.4608)
  line L96 (42.3963, -31.8564) -> (42.8322, -31.9465)
  line L97 (42.8322, -31.9465) -> (42.8322, -32.2329)
  line L98 (42.8322, -32.2329) -> (43.1801, -32.3046)
  line L99 (43.1801, -32.3046) -> (43.5853, -32.9778)
  line L100 (43.5853, -32.9778) -> (42.8322, -32.8203)
  line L101 (42.8322, -32.8203) -> (42.8322, -33.1784)
  line L102 (42.8322, -33.1784) -> (42.3963, -33.0883)
  line L103 (42.3963, -33.0883) -> (42.3963, -32.7282)
  line L104 (42.3963, -32.7282) -> (41.4857, -32.5379)
  spline S232 degree 2 poles (41.4857, -32.5379) (41.2381, -32.4867) (41.2033, -32.4867) knots 0 0 0 1 1 1
  spline S233 degree 2 poles (41.2033, -32.4867) (41.1357, -32.4867) (41.0979, -32.5297) knots 0 0 0 1 1 1
  spline S234 degree 2 poles (41.0979, -32.5297) (41.06, -32.5726) (41.06, -32.6852) knots 0 0 0 1 1 1
  spline S235 degree 2 poles (41.06, -32.6852) (41.06, -32.7241) (41.0744, -32.8796) knots 0 0 0 1 1 1
  line L105 (41.0744, -32.8796) -> (40.6385, -32.7875)
  spline S236 degree 2 poles (40.6385, -32.7875) (40.6078, -32.6361) (40.6078, -32.4765) knots 0 0 0 1 1 1
  spline S237 degree 2 poles (40.6078, -32.4765) (40.6078, -32.1654) (40.7275, -32.0242) knots 0 0 0 1 1 1
  spline S238 degree 2 poles (40.7275, -32.0242) (40.8472, -31.883) (41.06, -31.883) knots 0 0 0 1 1 1
  spline S239 degree 2 poles (41.06, -31.883) (41.1603, -31.883) (41.5225, -31.9587) knots 0 0 0 1 1 1
  line L106 (41.5225, -31.9587) -> (42.3963, -32.1409)
  line L107 (42.3963, -32.1409) -> (42.3963, -31.8564)
  line L108 (41.5634, -35.2207) -> (41.5634, -33.7473)
  spline S240 degree 2 poles (41.5634, -33.7473) (41.5287, -33.7452) (41.5102, -33.7452) knots 0 0 0 1 1 1
  spline S241 degree 2 poles (41.5102, -33.7452) (41.2933, -33.7452) (41.1603, -33.869) knots 0 0 0 1 1 1
  spline S242 degree 2 poles (41.1603, -33.869) (41.0273, -33.9928) (41.0273, -34.1709) knots 0 0 0 1 1 1
  spline S243 degree 2 poles (41.0273, -34.1709) (41.0273, -34.4635) (41.3302, -34.6272) knots 0 0 0 1 1 1
  line L109 (41.3302, -34.6272) -> (41.2422, -35.1531)
  spline S244 degree 2 poles (41.2422, -35.1531) (40.925, -34.9997) (40.7664, -34.7428) knots 0 0 0 1 1 1
  spline S245 degree 2 poles (40.7664, -34.7428) (40.6078, -34.486) (40.6078, -34.1668) knots 0 0 0 1 1 1
  spline S246 degree 2 poles (40.6078, -34.1668) (40.6078, -33.7289) (40.8851, -33.4546) knots 0 0 0 1 1 1
  spline S247 degree 2 poles (40.8851, -33.4546) (41.1623, -33.1804) (41.6187, -33.1804) knots 0 0 0 1 1 1
  spline S248 degree 2 poles (41.6187, -33.1804) (42.0648, -33.1804) (42.4127, -33.428) knots 0 0 0 1 1 1
  spline S249 degree 2 poles (42.4127, -33.428) (42.8834, -33.7657) (42.8834, -34.3919) knots 0 0 0 1 1 1
  spline S250 degree 2 poles (42.8834, -34.3919) (42.8834, -34.7909) (42.6368, -35.0263) knots 0 0 0 1 1 1
  spline S251 degree 2 poles (42.6368, -35.0263) (42.3902, -35.2616) (41.9461, -35.2616) knots 0 0 0 1 1 1
  spline S252 degree 2 poles (41.9461, -35.2616) (41.7333, -35.2616) (41.5634, -35.2207) knots 0 0 0 1 1 1
  spline S253 degree 2 poles (41.9216, -34.7254) (41.9604, -34.7275) (41.9809, -34.7275) knots 0 0 0 1 1 1
  spline S254 degree 2 poles (41.9809, -34.7275) (42.2224, -34.7275) (42.3431, -34.619) knots 0 0 0 1 1 1
  spline S255 degree 2 poles (42.3431, -34.619) (42.4638, -34.5106) (42.4638, -34.3284) knots 0 0 0 1 1 1
  spline S256 degree 2 poles (42.4638, -34.3284) (42.4638, -34.1463) (42.3267, -34.002) knots 0 0 0 1 1 1
  spline S257 degree 2 poles (42.3267, -34.002) (42.1896, -33.8578) (41.9216, -33.8066) knots 0 0 0 1 1 1
  line L110 (41.9216, -33.8066) -> (41.9216, -34.7254)
  line L111 (42.8322, -35.8571) -> (42.8322, -36.4055)
  line L112 (42.8322, -36.4055) -> (42.4106, -36.3175)
  spline S258 degree 2 poles (42.4106, -36.3175) (42.8834, -36.6245) (42.8834, -36.9826) knots 0 0 0 1 1 1
  spline S259 degree 2 poles (42.8834, -36.9826) (42.8834, -37.1095) (42.8199, -37.2548) knots 0 0 0 1 1 1
  line L113 (42.8199, -37.2548) -> (42.339, -37.0297)
  spline S260 degree 2 poles (42.339, -37.0297) (42.3677, -36.9499) (42.3677, -36.8598) knots 0 0 0 1 1 1
  spline S261 degree 2 poles (42.3677, -36.8598) (42.3677, -36.7084) (42.2531, -36.5518) knots 0 0 0 1 1 1
  spline S262 degree 2 poles (42.2531, -36.5518) (42.1385, -36.3953) (41.9471, -36.3073) knots 0 0 0 1 1 1
  spline S263 degree 2 poles (41.9471, -36.3073) (41.7558, -36.2193) (41.3404, -36.1334) knots 0 0 0 1 1 1
  line L114 (41.3404, -36.1334) -> (40.6589, -35.9901)
  line L115 (40.6589, -35.9901) -> (40.6589, -35.4028)
  line L116 (40.6589, -35.4028) -> (42.8322, -35.8571)
  line L117 (42.8322, -37.2486) -> (42.8322, -37.8339)
  line L118 (42.8322, -37.8339) -> (41.7497, -37.9812)
  spline S264 degree 2 poles (41.7497, -37.9812) (41.3322, -38.0365) (41.1644, -38.0426) knots 0 0 0 1 1 1
  spline S265 degree 2 poles (41.1644, -38.0426) (41.498, -38.1572) (41.8683, -38.3578) knots 0 0 0 1 1 1
  line L119 (41.8683, -38.3578) -> (42.8322, -38.8776)
  line L120 (42.8322, -38.8776) -> (42.8322, -39.4997)
  line L121 (42.8322, -39.4997) -> (40.4461, -38.1572)
  spline S266 degree 2 poles (40.4461, -38.1572) (40.1494, -37.9915) (40.0307, -37.8963) knots 0 0 0 1 1 1
  spline S267 degree 2 poles (40.0307, -37.8963) (39.912, -37.8012) (39.8445, -37.6671) knots 0 0 0 1 1 1
  spline S268 degree 2 poles (39.8445, -37.6671) (39.7769, -37.5331) (39.7769, -37.3448) knots 0 0 0 1 1 1
  spline S269 degree 2 poles (39.7769, -37.3448) (39.7769, -37.1586) (39.8424, -36.9253) knots 0 0 0 1 1 1
  line L122 (39.8424, -36.9253) -> (40.2804, -36.9765)
  spline S270 degree 2 poles (40.2804, -36.9765) (40.2497, -37.0829) (40.2497, -37.1832) knots 0 0 0 1 1 1
  spline S271 degree 2 poles (40.2497, -37.1832) (40.2497, -37.4533) (40.6589, -37.6272) knots 0 0 0 1 1 1
  line L123 (40.6589, -37.6272) -> (42.8322, -37.2486)
extrude "Extrude2" cut sketch "Sketch2" against normal blind 0.5 contours L4 S0 S1 S2 S3 S4 S5 S6 L5 S7 S8 S9 S10 S11 S12 S13 L6 S14 S15 S16 S17 S18 S19 S20 S21 S22 S23 S24 S25 | L7 L8 L9 L10 | L11 L12 L13 S26 S27 S28 S29 L14 S30 S31 S32 L15 | L16 L17 L18 L19 S33 S34 S35 L20 L21 L22 | L23 L24 S36 S37 L25 S38 S39 L26 L27 | L28 S40 L29 L30 L31 L32 S41 S42 | L33 S43 S44 S45 S46 S47 S48 S49 S50 S51 L34 L35 L36 S52 S53 S54 S55 S56 S57 S58 S59 S60 S61 | S62 S63 S64 S65 S66 S67 S68 S69 S70 S71 | L37 L38 S82 S83 S84 S85 S86 S87 S88 S89 L39 L40 L41 S90 S91 S92 S93 S94 L42 L43 L44 S95 S96 S97 S98 S99 S100 S101 L45 L46 L47 | L48 S102 S103 S104 S105 S106 S107 S108 S109 L49 S110 S111 S112 S113 S114 S115 S116 S117 S118 S119 S120 S121 S122 | L51 L52 L53 L54 S131 S132 S133 S134 S135 L55 L56 L57 S136 S137 S138 S139 S140 S141 L58 | L59 L60 L61 L62 | L63 L64 L65 L66 | L67 L68 L69 L70 | L71 L72 S142 S143 S144 S145 S146 S147 S148 L73 L74 L75 | S159 S160 S161 S162 S163 S164 S165 S166 S167 | L76 L77 L78 S177 S178 S179 S180 S181 S182 S183 S184 S185 L79 L80 | L81 S195 S196 S197 S198 S199 S200 S201 S202 L82 S203 S204 S205 S206 S207 S208 S209 S210 S211 S212 S213 S214 S215 | L84 L85 L86 L87 L88 L89 L90 L91 L92 S224 S225 S226 S227 L93 S228 S229 S230 S231 L94 L95 | L96 L97 L98 L99 L100 L101 L102 L103 L104 S232 S233 S234 S235 L105 S236 S237 S238 S239 L106 L107 | L108 S240 S241 S242 S243 L109 S244 S245 S246 S247 S248 S249 S250 S251 S252 | L111 L112 S258 S259 L113 S260 S261 S262 S263 L114 L115 L116 L123 | S259 L113 L117 L118 S264 S265 L119 L120 L121 S266 S267 S268 S269 L122 S270 S271 L123
